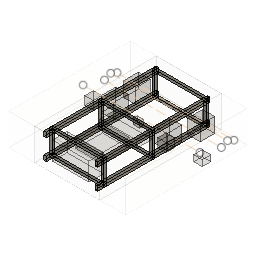
GP_TARS_V2_1000_CONCEPT_V0 (Autodesk Fusion 360 design; units mm, degrees)
part number: 2026-08-09-22-24-51-238
part number: 2026-08-09-22-24-51-360
part number: 2026-08-09-22-24-51-366
part number: 2026-08-09-22-24-51-368
part number: 2026-08-09-22-24-51-370
part number: 2026-08-09-22-24-51-373
part number: 2026-08-09-22-24-51-375
part number: 2026-08-09-22-24-51-377
part number: 2026-08-09-22-24-51-379
part number: 2026-08-09-22-24-51-381
part number: 2026-08-09-22-24-51-383
part number: 2026-08-09-22-24-51-385
part number: 2026-08-09-22-24-51-387
part number: 2026-08-09-22-24-51-390
part number: 2026-08-09-22-24-51-392
part number: 2026-08-09-22-24-51-395
part number: 2026-08-09-22-24-51-398
part number: 2026-08-09-22-24-51-400
part number: 2026-08-09-22-24-51-403
part number: 2026-08-09-22-24-51-405
part number: 2026-08-09-22-24-51-407
part number: 2026-08-09-22-24-51-410
part number: 2026-08-09-22-24-51-412
part number: 2026-08-09-22-24-51-415
part number: 2026-08-09-22-24-51-417
part number: 2026-08-09-22-24-51-420
part number: 2026-08-09-22-24-51-423
part number: 2026-08-09-22-24-51-426
part number: 2026-08-09-22-24-51-429
part number: 2026-08-09-22-24-51-432
part number: 2026-08-09-22-24-51-435
part number: 2026-08-09-22-24-51-438
part number: 2026-08-09-22-24-51-441
part number: 2026-08-09-22-24-51-444
part number: 2026-08-09-22-24-51-448
part number: 2026-08-09-22-24-51-451
part number: 2026-08-09-22-24-51-454
part number: 2026-08-09-22-24-51-459
part number: 2026-08-09-22-24-51-463
part number: 2026-08-09-22-24-51-467
part number: 2026-08-09-22-24-51-471
part number: 2026-08-09-22-24-51-475
part number: 2026-08-09-22-24-51-479
part number: 2026-08-09-22-24-51-483
part number: 2026-08-09-22-24-51-487
part number: 2026-08-09-22-24-51-492
part number: 2026-08-09-22-24-51-496
part number: 2026-08-09-22-24-51-501
part number: 2026-08-09-22-24-51-505
part number: 2026-08-09-22-24-51-510
part number: 2026-08-09-22-24-51-514
part number: 2026-08-09-22-24-51-519
part number: 2026-08-09-22-24-51-524
part number: 2026-08-09-22-24-51-612
part number: 2026-08-09-22-24-51-658
part number: 2026-08-09-22-24-51-683
part number: 2026-08-09-22-24-51-707
part number: 2026-08-09-22-24-51-732
part number: 2026-08-09-22-24-51-761
part number: 2026-08-09-22-24-51-801
part number: 2026-08-09-22-24-51-843
part number: 2026-08-09-22-24-51-883
part number: 2026-08-09-22-24-51-924
part number: 2026-08-09-22-24-51-965
part number: 2026-08-09-22-24-52-009
part number: 2026-08-09-22-24-52-056
part number: 2026-08-09-22-24-52-102
part number: 2026-08-09-22-24-52-148
part number: 2026-08-09-22-24-52-195
part number: 2026-08-09-22-24-52-243
part number: 2026-08-09-22-24-52-292
part number: 2026-08-09-22-24-52-342
part number: 2026-08-09-22-24-52-394
part number: 2026-08-09-22-24-52-450
part number: 2026-08-09-22-24-52-513
part number: 2026-08-09-22-24-52-576
part number: 2026-08-09-22-24-52-637
part number: 2026-08-09-22-24-52-701
part number: 2026-08-09-22-24-52-761
part number: 2026-08-09-22-24-52-825
part number: 2026-08-09-22-24-52-889
part number: 2026-08-09-22-24-52-958
part number: 2026-08-09-22-24-53-024
part number: 2026-08-09-22-24-53-092
part number: 2026-08-09-22-24-53-162
Autodesk Fusion 360 part; units mm, degrees
sketch "EXTERNAL_REFERENCE_ENVELOPE_PROFILE" plane through (0, 0, 0) normal (0, 0, 1) x (1, 0, 0) in component "EXTERNAL_REFERENCE_ENVELOPE"
  line L0 (-479.3589, 0) -> (479.3589, 0)
  line L1 (479.3589, 0) -> (479.3589, 1000)
  line L2 (479.3589, 1000) -> (-479.3589, 1000)
  line L3 (-479.3589, 1000) -> (-479.3589, 0)
extrude "Extrude1" add sketch "EXTERNAL_REFERENCE_ENVELOPE_PROFILE" along normal blind 259.8674 makes body 1 in component "EXTERNAL_REFERENCE_ENVELOPE"
move_body "Move1" bodies 1 to x (1, 0, 0) y (0, 1, 0) z (0, 0, 1) at (0, 0, -129.9337) in component "EXTERNAL_REFERENCE_ENVELOPE"
sketch "CENTRAL_CHASSIS_REFERENCE_PROFILE" plane through (0, 0, 0) normal (0, 0, 1) x (1, 0, 0) in component "CENTRAL_CHASSIS_REFERENCE"
  line L0 (-266.0414, 0) -> (266.0414, 0)
  line L1 (266.0414, 0) -> (266.0414, 998.6144)
  line L2 (266.0414, 998.6144) -> (-266.0414, 998.6144)
  line L3 (-266.0414, 998.6144) -> (-266.0414, 0)
extrude "Extrude1'" add sketch "CENTRAL_CHASSIS_REFERENCE_PROFILE" along normal blind 259.8674 separate body makes body 2 in component "CENTRAL_CHASSIS_REFERENCE"
move_body "Move1'" bodies 2 to x (1, 0, 0) y (0, 1, 0) z (0, 0, 1) at (0, 0, -129.9337) in component "CENTRAL_CHASSIS_REFERENCE"
ref_plane "WorkPlane1" through (0, 0, 0) normal (1, 0, 0) x (0, 1, 0) in component "DATUMS"
ref_plane "WorkPlane2" through (0, 0, 0) normal (0, 1, 0) x (0, 0, 1) in component "DATUMS"
ref_plane "WorkPlane3" through (0, 0, 0) normal (0, 0, 1) x (1, 0, 0) in component "DATUMS"
ref_plane "WorkPlane1" through (0, 0, -19.948) normal (0, 0, 1) x (1, 0, 0) in component "JOINT_UPPER_MAIN_REF"
sketch "JOINT_UPPER_MAIN_REF_AXIS_X" plane through (0, 0, -19.948) normal (0, 0, 1) x (1, 0, 0) in component "JOINT_UPPER_MAIN_REF"
  line L0 (-479.3589, 837.977) -> (479.3589, 837.977) construction
ref_plane "WorkPlane1" through (0, 0, -41.913) normal (0, 0, 1) x (1, 0, 0) in component "JOINT_UPPER_SECONDARY_REF"
sketch "JOINT_UPPER_SECONDARY_REF_AXIS_X" plane through (0, 0, -41.913) normal (0, 0, 1) x (1, 0, 0) in component "JOINT_UPPER_SECONDARY_REF"
  line L0 (-479.3589, 889.895) -> (479.3589, 889.895) construction
ref_plane "WorkPlane1" through (0, 0, -41.913) normal (0, 0, 1) x (1, 0, 0) in component "JOINT_LOWER_SECONDARY_REF"
sketch "JOINT_LOWER_SECONDARY_REF_AXIS_X" plane through (0, 0, -41.913) normal (0, 0, 1) x (1, 0, 0) in component "JOINT_LOWER_SECONDARY_REF"
  line L0 (-479.3589, 786.06) -> (479.3589, 786.06) construction
ref_plane "WorkPlane1" through (0, 0, 10.004) normal (0, 0, 1) x (1, 0, 0) in component "JOINT_LOWER_MAIN_REF"
sketch "JOINT_LOWER_MAIN_REF_AXIS_X" plane through (0, 0, 10.004) normal (0, 0, 1) x (1, 0, 0) in component "JOINT_LOWER_MAIN_REF"
  line L0 (-479.3589, 610.838) -> (479.3589, 610.838) construction
sketch "FRAME_VERTICAL_0_0_PROFILE" plane through (0, 0, 0) normal (0, 0, 1) x (1, 0, 0) in component "FRAME_VERTICAL_0_0"
  line L0 (-220, 30) -> (-200, 30)
  line L1 (-200, 30) -> (-200, 950)
  line L2 (-200, 950) -> (-220, 950)
  line L3 (-220, 950) -> (-220, 30)
extrude "Extrude1''" add sketch "FRAME_VERTICAL_0_0_PROFILE" along normal blind 40 separate body makes body 3 in component "FRAME_VERTICAL_0_0"
move_body "Move1''" bodies 3 to x (1, 0, 0) y (0, 1, 0) z (0, 0, 1) at (0, 0, -105) in component "FRAME_VERTICAL_0_0"
sketch "FRAME_VERTICAL_0_1_PROFILE" plane through (0, 0, 0) normal (0, 0, 1) x (1, 0, 0) in component "FRAME_VERTICAL_0_1"
  line L0 (-220, 30) -> (-200, 30)
  line L1 (-200, 30) -> (-200, 950)
  line L2 (-200, 950) -> (-220, 950)
  line L3 (-220, 950) -> (-220, 30)
extrude "Extrude1'''" add sketch "FRAME_VERTICAL_0_1_PROFILE" along normal blind 40 separate body makes body 4 in component "FRAME_VERTICAL_0_1"
move_body "Move1'''" bodies 4 to x (1, 0, 0) y (0, 1, 0) z (0, 0, 1) at (0, 0, 65) in component "FRAME_VERTICAL_0_1"
sketch "FRAME_VERTICAL_1_0_PROFILE" plane through (0, 0, 0) normal (0, 0, 1) x (1, 0, 0) in component "FRAME_VERTICAL_1_0"
  line L0 (200, 30) -> (220, 30)
  line L1 (220, 30) -> (220, 950)
  line L2 (220, 950) -> (200, 950)
  line L3 (200, 950) -> (200, 30)
extrude "Extrude1''''" add sketch "FRAME_VERTICAL_1_0_PROFILE" along normal blind 40 separate body makes body 5 in component "FRAME_VERTICAL_1_0"
move_body "Move1''''" bodies 5 to x (1, 0, 0) y (0, 1, 0) z (0, 0, 1) at (0, 0, -105) in component "FRAME_VERTICAL_1_0"
sketch "FRAME_VERTICAL_1_1_PROFILE" plane through (0, 0, 0) normal (0, 0, 1) x (1, 0, 0) in component "FRAME_VERTICAL_1_1"
  line L0 (200, 30) -> (220, 30)
  line L1 (220, 30) -> (220, 950)
  line L2 (220, 950) -> (200, 950)
  line L3 (200, 950) -> (200, 30)
extrude "Extrude1'''''" add sketch "FRAME_VERTICAL_1_1_PROFILE" along normal blind 40 separate body makes body 6 in component "FRAME_VERTICAL_1_1"
move_body "Move1'''''" bodies 6 to x (1, 0, 0) y (0, 1, 0) z (0, 0, 1) at (0, 0, 65) in component "FRAME_VERTICAL_1_1"
sketch "FRAME_CROSS_LOW_FRONT_PROFILE" plane through (0, 0, 0) normal (0, 0, 1) x (1, 0, 0) in component "FRAME_CROSS_LOW_FRONT"
  line L0 (-220, 80) -> (220, 80)
  line L1 (220, 80) -> (220, 100)
  line L2 (220, 100) -> (-220, 100)
  line L3 (-220, 100) -> (-220, 80)
extrude "Extrude1''''''" add sketch "FRAME_CROSS_LOW_FRONT_PROFILE" along normal blind 20 separate body makes body 7 in component "FRAME_CROSS_LOW_FRONT"
move_body "Move1''''''" bodies 7 to x (1, 0, 0) y (0, 1, 0) z (0, 0, 1) at (0, 0, -105) in component "FRAME_CROSS_LOW_FRONT"
sketch "FRAME_CROSS_LOW_REAR_PROFILE" plane through (0, 0, 0) normal (0, 0, 1) x (1, 0, 0) in component "FRAME_CROSS_LOW_REAR"
  line L0 (-220, 80) -> (220, 80)
  line L1 (220, 80) -> (220, 100)
  line L2 (220, 100) -> (-220, 100)
  line L3 (-220, 100) -> (-220, 80)
extrude "Extrude1'''''''" add sketch "FRAME_CROSS_LOW_REAR_PROFILE" along normal blind 20 separate body makes body 8 in component "FRAME_CROSS_LOW_REAR"
move_body "Move1'''''''" bodies 8 to x (1, 0, 0) y (0, 1, 0) z (0, 0, 1) at (0, 0, 85) in component "FRAME_CROSS_LOW_REAR"
sketch "FRAME_DEPTH_LOW_LEFT_PROFILE" plane through (0, 0, 0) normal (0, 0, 1) x (1, 0, 0) in component "FRAME_DEPTH_LOW_LEFT"
  line L0 (-220, 80) -> (-200, 80)
  line L1 (-200, 80) -> (-200, 100)
  line L2 (-200, 100) -> (-220, 100)
  line L3 (-220, 100) -> (-220, 80)
extrude "Extrude1''''''''" add sketch "FRAME_DEPTH_LOW_LEFT_PROFILE" along normal blind 170 separate body makes body 9 in component "FRAME_DEPTH_LOW_LEFT"
move_body "Move1''''''''" bodies 9 to x (1, 0, 0) y (0, 1, 0) z (0, 0, 1) at (0, 0, -85) in component "FRAME_DEPTH_LOW_LEFT"
sketch "FRAME_DEPTH_LOW_RIGHT_PROFILE" plane through (0, 0, 0) normal (0, 0, 1) x (1, 0, 0) in component "FRAME_DEPTH_LOW_RIGHT"
  line L0 (200, 80) -> (220, 80)
  line L1 (220, 80) -> (220, 100)
  line L2 (220, 100) -> (200, 100)
  line L3 (200, 100) -> (200, 80)
extrude "Extrude1'''''''''" add sketch "FRAME_DEPTH_LOW_RIGHT_PROFILE" along normal blind 170 separate body makes body 10 in component "FRAME_DEPTH_LOW_RIGHT"
move_body "Move1'''''''''" bodies 10 to x (1, 0, 0) y (0, 1, 0) z (0, 0, 1) at (0, 0, -85) in component "FRAME_DEPTH_LOW_RIGHT"
sketch "FRAME_CROSS_MID_FRONT_PROFILE" plane through (0, 0, 0) normal (0, 0, 1) x (1, 0, 0) in component "FRAME_CROSS_MID_FRONT"
  line L0 (-220, 480) -> (220, 480)
  line L1 (220, 480) -> (220, 500)
  line L2 (220, 500) -> (-220, 500)
  line L3 (-220, 500) -> (-220, 480)
extrude "Extrude1''''''''''" add sketch "FRAME_CROSS_MID_FRONT_PROFILE" along normal blind 20 separate body makes body 11 in component "FRAME_CROSS_MID_FRONT"
move_body "Move1''''''''''" bodies 11 to x (1, 0, 0) y (0, 1, 0) z (0, 0, 1) at (0, 0, -105) in component "FRAME_CROSS_MID_FRONT"
sketch "FRAME_CROSS_MID_REAR_PROFILE" plane through (0, 0, 0) normal (0, 0, 1) x (1, 0, 0) in component "FRAME_CROSS_MID_REAR"
  line L0 (-220, 480) -> (220, 480)
  line L1 (220, 480) -> (220, 500)
  line L2 (220, 500) -> (-220, 500)
  line L3 (-220, 500) -> (-220, 480)
extrude "Extrude1'''''''''''" add sketch "FRAME_CROSS_MID_REAR_PROFILE" along normal blind 20 separate body makes body 12 in component "FRAME_CROSS_MID_REAR"
move_body "Move1'''''''''''" bodies 12 to x (1, 0, 0) y (0, 1, 0) z (0, 0, 1) at (0, 0, 85) in component "FRAME_CROSS_MID_REAR"
sketch "FRAME_DEPTH_MID_LEFT_PROFILE" plane through (0, 0, 0) normal (0, 0, 1) x (1, 0, 0) in component "FRAME_DEPTH_MID_LEFT"
  line L0 (-220, 480) -> (-200, 480)
  line L1 (-200, 480) -> (-200, 500)
  line L2 (-200, 500) -> (-220, 500)
  line L3 (-220, 500) -> (-220, 480)
extrude "Extrude1''''''''''''" add sketch "FRAME_DEPTH_MID_LEFT_PROFILE" along normal blind 170 separate body makes body 13 in component "FRAME_DEPTH_MID_LEFT"
move_body "Move1''''''''''''" bodies 13 to x (1, 0, 0) y (0, 1, 0) z (0, 0, 1) at (0, 0, -85) in component "FRAME_DEPTH_MID_LEFT"
sketch "FRAME_DEPTH_MID_RIGHT_PROFILE" plane through (0, 0, 0) normal (0, 0, 1) x (1, 0, 0) in component "FRAME_DEPTH_MID_RIGHT"
  line L0 (200, 480) -> (220, 480)
  line L1 (220, 480) -> (220, 500)
  line L2 (220, 500) -> (200, 500)
  line L3 (200, 500) -> (200, 480)
extrude "Extrude1'''''''''''''" add sketch "FRAME_DEPTH_MID_RIGHT_PROFILE" along normal blind 170 separate body makes body 14 in component "FRAME_DEPTH_MID_RIGHT"
move_body "Move1'''''''''''''" bodies 14 to x (1, 0, 0) y (0, 1, 0) z (0, 0, 1) at (0, 0, -85) in component "FRAME_DEPTH_MID_RIGHT"
sketch "FRAME_CROSS_HIGH_FRONT_PROFILE" plane through (0, 0, 0) normal (0, 0, 1) x (1, 0, 0) in component "FRAME_CROSS_HIGH_FRONT"
  line L0 (-220, 920) -> (220, 920)
  line L1 (220, 920) -> (220, 940)
  line L2 (220, 940) -> (-220, 940)
  line L3 (-220, 940) -> (-220, 920)
extrude "Extrude1''''''''''''''" add sketch "FRAME_CROSS_HIGH_FRONT_PROFILE" along normal blind 20 separate body makes body 15 in component "FRAME_CROSS_HIGH_FRONT"
move_body "Move1''''''''''''''" bodies 15 to x (1, 0, 0) y (0, 1, 0) z (0, 0, 1) at (0, 0, -105) in component "FRAME_CROSS_HIGH_FRONT"
sketch "FRAME_CROSS_HIGH_REAR_PROFILE" plane through (0, 0, 0) normal (0, 0, 1) x (1, 0, 0) in component "FRAME_CROSS_HIGH_REAR"
  line L0 (-220, 920) -> (220, 920)
  line L1 (220, 920) -> (220, 940)
  line L2 (220, 940) -> (-220, 940)
  line L3 (-220, 940) -> (-220, 920)
extrude "Extrude1'''''''''''''''" add sketch "FRAME_CROSS_HIGH_REAR_PROFILE" along normal blind 20 separate body makes body 16 in component "FRAME_CROSS_HIGH_REAR"
move_body "Move1'''''''''''''''" bodies 16 to x (1, 0, 0) y (0, 1, 0) z (0, 0, 1) at (0, 0, 85) in component "FRAME_CROSS_HIGH_REAR"
sketch "FRAME_DEPTH_HIGH_LEFT_PROFILE" plane through (0, 0, 0) normal (0, 0, 1) x (1, 0, 0) in component "FRAME_DEPTH_HIGH_LEFT"
  line L0 (-220, 920) -> (-200, 920)
  line L1 (-200, 920) -> (-200, 940)
  line L2 (-200, 940) -> (-220, 940)
  line L3 (-220, 940) -> (-220, 920)
extrude "Extrude1''''''''''''''''" add sketch "FRAME_DEPTH_HIGH_LEFT_PROFILE" along normal blind 170 separate body makes body 17 in component "FRAME_DEPTH_HIGH_LEFT"
move_body "Move1''''''''''''''''" bodies 17 to x (1, 0, 0) y (0, 1, 0) z (0, 0, 1) at (0, 0, -85) in component "FRAME_DEPTH_HIGH_LEFT"
sketch "FRAME_DEPTH_HIGH_RIGHT_PROFILE" plane through (0, 0, 0) normal (0, 0, 1) x (1, 0, 0) in component "FRAME_DEPTH_HIGH_RIGHT"
  line L0 (200, 920) -> (220, 920)
  line L1 (220, 920) -> (220, 940)
  line L2 (220, 940) -> (200, 940)
  line L3 (200, 940) -> (200, 920)
extrude "Extrude1'''''''''''''''''" add sketch "FRAME_DEPTH_HIGH_RIGHT_PROFILE" along normal blind 170 separate body makes body 18 in component "FRAME_DEPTH_HIGH_RIGHT"
move_body "Move1'''''''''''''''''" bodies 18 to x (1, 0, 0) y (0, 1, 0) z (0, 0, 1) at (0, 0, -85) in component "FRAME_DEPTH_HIGH_RIGHT"
sketch "BATTERY_KEEP_OUT_PROFILE" plane through (0, 0, 0) normal (0, 0, 1) x (1, 0, 0) in component "BATTERY_KEEP_OUT"
  line L0 (-150, 30) -> (150, 30)
  line L1 (150, 30) -> (150, 150)
  line L2 (150, 150) -> (-150, 150)
  line L3 (-150, 150) -> (-150, 30)
extrude "Extrude1''''''''''''''''''" add sketch "BATTERY_KEEP_OUT_PROFILE" along normal blind 150 separate body makes body 19 in component "BATTERY_KEEP_OUT"
move_body "Move1''''''''''''''''''" bodies 19 to x (1, 0, 0) y (0, 1, 0) z (0, 0, 1) at (0, 0, -75) in component "BATTERY_KEEP_OUT"
sketch "MINI_PC_KEEP_OUT_PROFILE" plane through (0, 0, 0) normal (0, 0, 1) x (1, 0, 0) in component "MINI_PC_KEEP_OUT"
  line L0 (-110, 180) -> (110, 180)
  line L1 (110, 180) -> (110, 400)
  line L2 (110, 400) -> (-110, 400)
  line L3 (-110, 400) -> (-110, 180)
extrude "Extrude1'''''''''''''''''''" add sketch "MINI_PC_KEEP_OUT_PROFILE" along normal blind 80 separate body makes body 20 in component "MINI_PC_KEEP_OUT"
move_body "Move1'''''''''''''''''''" bodies 20 to x (1, 0, 0) y (0, 1, 0) z (0, 0, 1) at (0, 0, -40) in component "MINI_PC_KEEP_OUT"
sketch "GPU_KEEP_OUT_PROFILE" plane through (0, 0, 0) normal (0, 0, 1) x (1, 0, 0) in component "GPU_KEEP_OUT"
  line L0 (-150, 420) -> (150, 420)
  line L1 (150, 420) -> (150, 550)
  line L2 (150, 550) -> (-150, 550)
  line L3 (-150, 550) -> (-150, 420)
extrude "Extrude1''''''''''''''''''''" add sketch "GPU_KEEP_OUT_PROFILE" along normal blind 60 separate body makes body 21 in component "GPU_KEEP_OUT"
move_body "Move1''''''''''''''''''''" bodies 21 to x (1, 0, 0) y (0, 1, 0) z (0, 0, 1) at (0, 0, -30) in component "GPU_KEEP_OUT"
sketch "ACTUATOR_MAIN_UPPER_PORT_KEEP_OUT_PROFILE" plane through (0, 0, 0) normal (0, 0, 1) x (1, 0, 0) in component "ACTUATOR_MAIN_UPPER_PORT_KEEP_OUT"
  line L0 (214.041, 777.973) -> (314.041, 777.973)
  line L1 (314.041, 777.973) -> (314.041, 897.973)
  line L2 (314.041, 897.973) -> (214.041, 897.973)
  line L3 (214.041, 897.973) -> (214.041, 777.973)
extrude "Extrude1'''''''''''''''''''''" add sketch "ACTUATOR_MAIN_UPPER_PORT_KEEP_OUT_PROFILE" along normal blind 120 separate body makes body 22 in component "ACTUATOR_MAIN_UPPER_PORT_KEEP_OUT"
move_body "Move1'''''''''''''''''''''" bodies 22 to x (1, 0, 0) y (0, 1, 0) z (0, 0, 1) at (0, 0, -79.977) in component "ACTUATOR_MAIN_UPPER_PORT_KEEP_OUT"
sketch "ACTUATOR_MAIN_UPPER_STARBOARD_KEEP_OUT_PROFILE" plane through (0, 0, 0) normal (0, 0, 1) x (1, 0, 0) in component "ACTUATOR_MAIN_UPPER_STARBOARD_KEEP_OUT"
  line L0 (-314.041, 777.973) -> (-214.041, 777.973)
  line L1 (-214.041, 777.973) -> (-214.041, 897.973)
  line L2 (-214.041, 897.973) -> (-314.041, 897.973)
  line L3 (-314.041, 897.973) -> (-314.041, 777.973)
extrude "Extrude1''''''''''''''''''''''" add sketch "ACTUATOR_MAIN_UPPER_STARBOARD_KEEP_OUT_PROFILE" along normal blind 120 separate body makes body 23 in component "ACTUATOR_MAIN_UPPER_STARBOARD_KEEP_OUT"
move_body "Move1''''''''''''''''''''''" bodies 23 to x (1, 0, 0) y (0, 1, 0) z (0, 0, 1) at (0, 0, -79.977) in component "ACTUATOR_MAIN_UPPER_STARBOARD_KEEP_OUT"
sketch "ACTUATOR_MAIN_LOWER_PORT_KEEP_OUT_PROFILE" plane through (0, 0, 0) normal (0, 0, 1) x (1, 0, 0) in component "ACTUATOR_MAIN_LOWER_PORT_KEEP_OUT"
  line L0 (170, 550.838) -> (270, 550.838)
  line L1 (270, 550.838) -> (270, 670.838)
  line L2 (270, 670.838) -> (170, 670.838)
  line L3 (170, 670.838) -> (170, 550.838)
extrude "Extrude1'''''''''''''''''''''''" add sketch "ACTUATOR_MAIN_LOWER_PORT_KEEP_OUT_PROFILE" along normal blind 120 separate body makes body 24 in component "ACTUATOR_MAIN_LOWER_PORT_KEEP_OUT"
move_body "Move1'''''''''''''''''''''''" bodies 24 to x (1, 0, 0) y (0, 1, 0) z (0, 0, 1) at (0, 0, -49.996) in component "ACTUATOR_MAIN_LOWER_PORT_KEEP_OUT"
sketch "ACTUATOR_MAIN_LOWER_STARBOARD_KEEP_OUT_PROFILE" plane through (0, 0, 0) normal (0, 0, 1) x (1, 0, 0) in component "ACTUATOR_MAIN_LOWER_STARBOARD_KEEP_OUT"
  line L0 (-270, 550.838) -> (-170, 550.838)
  line L1 (-170, 550.838) -> (-170, 670.838)
  line L2 (-170, 670.838) -> (-270, 670.838)
  line L3 (-270, 670.838) -> (-270, 550.838)
extrude "Extrude1''''''''''''''''''''''''" add sketch "ACTUATOR_MAIN_LOWER_STARBOARD_KEEP_OUT_PROFILE" along normal blind 120 separate body makes body 25 in component "ACTUATOR_MAIN_LOWER_STARBOARD_KEEP_OUT"
move_body "Move1''''''''''''''''''''''''" bodies 25 to x (1, 0, 0) y (0, 1, 0) z (0, 0, 1) at (0, 0, -49.996) in component "ACTUATOR_MAIN_LOWER_STARBOARD_KEEP_OUT"
sketch "ACTUATOR_SECONDARY_PORT_KEEP_OUT_PROFILE" plane through (0, 0, 0) normal (0, 0, 1) x (1, 0, 0) in component "ACTUATOR_SECONDARY_PORT_KEEP_OUT"
  line L0 (264.185, 479.664) -> (334.185, 479.664)
  line L1 (334.185, 479.664) -> (334.185, 549.664)
  line L2 (334.185, 549.664) -> (264.185, 549.664)
  line L3 (264.185, 549.664) -> (264.185, 479.664)
extrude "Extrude1'''''''''''''''''''''''''" add sketch "ACTUATOR_SECONDARY_PORT_KEEP_OUT_PROFILE" along normal blind 70 separate body makes body 26 in component "ACTUATOR_SECONDARY_PORT_KEEP_OUT"
move_body "Move1'''''''''''''''''''''''''" bodies 26 to x (1, 0, 0) y (0, 1, 0) z (0, 0, 1) at (0, 0, 2.955) in component "ACTUATOR_SECONDARY_PORT_KEEP_OUT"
sketch "ACTUATOR_SECONDARY_STARBOARD_KEEP_OUT_PROFILE" plane through (0, 0, 0) normal (0, 0, 1) x (1, 0, 0) in component "ACTUATOR_SECONDARY_STARBOARD_KEEP_OUT"
  line L0 (-334.185, 479.664) -> (-264.185, 479.664)
  line L1 (-264.185, 479.664) -> (-264.185, 549.664)
  line L2 (-264.185, 549.664) -> (-334.185, 549.664)
  line L3 (-334.185, 549.664) -> (-334.185, 479.664)
extrude "Extrude1''''''''''''''''''''''''''" add sketch "ACTUATOR_SECONDARY_STARBOARD_KEEP_OUT_PROFILE" along normal blind 70 separate body makes body 27 in component "ACTUATOR_SECONDARY_STARBOARD_KEEP_OUT"
move_body "Move1''''''''''''''''''''''''''" bodies 27 to x (1, 0, 0) y (0, 1, 0) z (0, 0, 1) at (0, 0, 2.955) in component "ACTUATOR_SECONDARY_STARBOARD_KEEP_OUT"
sketch "E_STOP_KEEP_OUT_PROFILE" plane through (0, 0, 0) normal (0, 0, 1) x (1, 0, 0) in component "E_STOP_KEEP_OUT"
  line L0 (389.3589, 650) -> (459.3589, 650)
  line L1 (459.3589, 650) -> (459.3589, 720)
  line L2 (459.3589, 720) -> (389.3589, 720)
  line L3 (389.3589, 720) -> (389.3589, 650)
extrude "Extrude1'''''''''''''''''''''''''''" add sketch "E_STOP_KEEP_OUT_PROFILE" along normal blind 50 separate body makes body 28 in component "E_STOP_KEEP_OUT"
move_body "Move1'''''''''''''''''''''''''''" bodies 28 to x (1, 0, 0) y (0, 1, 0) z (0, 0, 1) at (0, 0, -119.9337) in component "E_STOP_KEEP_OUT"
sketch "IMU_KEEP_OUT_PROFILE" plane through (0, 0, 0) normal (0, 0, 1) x (1, 0, 0) in component "IMU_KEEP_OUT"
  line L0 (-25, 570) -> (25, 570)
  line L1 (25, 570) -> (25, 600)
  line L2 (25, 600) -> (-25, 600)
  line L3 (-25, 600) -> (-25, 570)
extrude "Extrude1''''''''''''''''''''''''''''" add sketch "IMU_KEEP_OUT_PROFILE" along normal blind 50 separate body makes body 29 in component "IMU_KEEP_OUT"
move_body "Move1''''''''''''''''''''''''''''" bodies 29 to x (1, 0, 0) y (0, 1, 0) z (0, 0, 1) at (0, 0, -25) in component "IMU_KEEP_OUT"
component "00_MASTER_REFERENCE" placed x (1, 0, 0) y (0, 1, 0) z (0, 0, 1) at (0, 0, 0)
component "01_FRAME" placed x (1, 0, 0) y (0, 1, 0) z (0, 0, 1) at (0, 0, 0)
component "02_JOINTS" placed x (1, 0, 0) y (0, 1, 0) z (0, 0, 1) at (0, 0, 0)
component "03_ACTUATORS" placed x (1, 0, 0) y (0, 1, 0) z (0, 0, 1) at (0, 0, 0)
component "04_BEARINGS_SHAFTS" placed x (1, 0, 0) y (0, 1, 0) z (0, 0, 1) at (0, 0, 0)
component "05_BATTERY" placed x (1, 0, 0) y (0, 1, 0) z (0, 0, 1) at (0, 0, 0)
component "06_COMPUTE" placed x (1, 0, 0) y (0, 1, 0) z (0, 0, 1) at (0, 0, 0)
component "07_GPU" placed x (1, 0, 0) y (0, 1, 0) z (0, 0, 1) at (0, 0, 0)
component "08_ELECTRONICS" placed x (1, 0, 0) y (0, 1, 0) z (0, 0, 1) at (0, 0, 0)
component "09_COOLING" placed x (1, 0, 0) y (0, 1, 0) z (0, 0, 1) at (0, 0, 0)
component "10_SENSORS" placed x (1, 0, 0) y (0, 1, 0) z (0, 0, 1) at (0, 0, 0)
component "11_BODY_PANELS" placed x (1, 0, 0) y (0, 1, 0) z (0, 0, 1) at (0, 0, 0)
component "12_FASTENERS" placed x (1, 0, 0) y (0, 1, 0) z (0, 0, 1) at (0, 0, 0)
component "13_WIRING" placed x (1, 0, 0) y (0, 1, 0) z (0, 0, 1) at (0, 0, 0)
component "Original_1000mm_Scaled_Geometry" placed x (1, 0, 0) y (0, 1, 0) z (0, 0, 1) at (0, 0, 0) in component "00_MASTER_REFERENCE"
component "DATUMS" placed x (1, 0, 0) y (0, 1, 0) z (0, 0, 1) at (0, 0, 0) in component "00_MASTER_REFERENCE"
component "Central_Spine" placed x (1, 0, 0) y (0, 1, 0) z (0, 0, 1) at (0, 0, 0) in component "01_FRAME"
component "Left_Frame" placed x (1, 0, 0) y (0, 1, 0) z (0, 0, 1) at (0, 0, 0) in component "01_FRAME"
component "Right_Frame" placed x (1, 0, 0) y (0, 1, 0) z (0, 0, 1) at (0, 0, 0) in component "01_FRAME"
component "Crossmembers" placed x (1, 0, 0) y (0, 1, 0) z (0, 0, 1) at (0, 0, 0) in component "01_FRAME"
component "FRAME_VERTICAL_0_0" placed x (1, 0, 0) y (0, 1, 0) z (0, 0, 1) at (0, 0, 0) in component "01_FRAME"
component "FRAME_VERTICAL_0_1" placed x (1, 0, 0) y (0, 1, 0) z (0, 0, 1) at (0, 0, 0) in component "01_FRAME"
component "FRAME_VERTICAL_1_0" placed x (1, 0, 0) y (0, 1, 0) z (0, 0, 1) at (0, 0, 0) in component "01_FRAME"
component "FRAME_VERTICAL_1_1" placed x (1, 0, 0) y (0, 1, 0) z (0, 0, 1) at (0, 0, 0) in component "01_FRAME"
component "FRAME_CROSS_LOW_FRONT" placed x (1, 0, 0) y (0, 1, 0) z (0, 0, 1) at (0, 0, 0) in component "01_FRAME"
component "FRAME_CROSS_LOW_REAR" placed x (1, 0, 0) y (0, 1, 0) z (0, 0, 1) at (0, 0, 0) in component "01_FRAME"
component "FRAME_DEPTH_LOW_LEFT" placed x (1, 0, 0) y (0, 1, 0) z (0, 0, 1) at (0, 0, 0) in component "01_FRAME"
component "FRAME_DEPTH_LOW_RIGHT" placed x (1, 0, 0) y (0, 1, 0) z (0, 0, 1) at (0, 0, 0) in component "01_FRAME"
component "FRAME_CROSS_MID_FRONT" placed x (1, 0, 0) y (0, 1, 0) z (0, 0, 1) at (0, 0, 0) in component "01_FRAME"
component "FRAME_CROSS_MID_REAR" placed x (1, 0, 0) y (0, 1, 0) z (0, 0, 1) at (0, 0, 0) in component "01_FRAME"
component "FRAME_DEPTH_MID_LEFT" placed x (1, 0, 0) y (0, 1, 0) z (0, 0, 1) at (0, 0, 0) in component "01_FRAME"
component "FRAME_DEPTH_MID_RIGHT" placed x (1, 0, 0) y (0, 1, 0) z (0, 0, 1) at (0, 0, 0) in component "01_FRAME"
component "FRAME_CROSS_HIGH_FRONT" placed x (1, 0, 0) y (0, 1, 0) z (0, 0, 1) at (0, 0, 0) in component "01_FRAME"
component "FRAME_CROSS_HIGH_REAR" placed x (1, 0, 0) y (0, 1, 0) z (0, 0, 1) at (0, 0, 0) in component "01_FRAME"
component "FRAME_DEPTH_HIGH_LEFT" placed x (1, 0, 0) y (0, 1, 0) z (0, 0, 1) at (0, 0, 0) in component "01_FRAME"
component "FRAME_DEPTH_HIGH_RIGHT" placed x (1, 0, 0) y (0, 1, 0) z (0, 0, 1) at (0, 0, 0) in component "01_FRAME"
component "Upper_Pivot" placed x (1, 0, 0) y (0, 1, 0) z (0, 0, 1) at (0, 0, 0) in component "02_JOINTS"
component "Lower_Pivot" placed x (1, 0, 0) y (0, 1, 0) z (0, 0, 1) at (0, 0, 0) in component "02_JOINTS"
component "Left_Leg_Pivot" placed x (1, 0, 0) y (0, 1, 0) z (0, 0, 1) at (0, 0, 0) in component "02_JOINTS"
component "Right_Leg_Pivot" placed x (1, 0, 0) y (0, 1, 0) z (0, 0, 1) at (0, 0, 0) in component "02_JOINTS"
component "JOINT_UPPER_MAIN_REF" placed x (1, 0, 0) y (0, 1, 0) z (0, 0, 1) at (0, 0, 0) in component "02_JOINTS"
component "JOINT_UPPER_SECONDARY_REF" placed x (1, 0, 0) y (0, 1, 0) z (0, 0, 1) at (0, 0, 0) in component "02_JOINTS"
component "JOINT_LOWER_SECONDARY_REF" placed x (1, 0, 0) y (0, 1, 0) z (0, 0, 1) at (0, 0, 0) in component "02_JOINTS"
component "JOINT_LOWER_MAIN_REF" placed x (1, 0, 0) y (0, 1, 0) z (0, 0, 1) at (0, 0, 0) in component "02_JOINTS"
component "ACTUATOR_MAIN_PLACEHOLDERS" placed x (1, 0, 0) y (0, 1, 0) z (0, 0, 1) at (0, 0, 0) in component "03_ACTUATORS"
component "ACTUATOR_SECONDARY_PLACEHOLDERS" placed x (1, 0, 0) y (0, 1, 0) z (0, 0, 1) at (0, 0, 0) in component "03_ACTUATORS"
component "ACTUATOR_MAIN_UPPER_PORT_KEEP_OUT" placed x (1, 0, 0) y (0, 1, 0) z (0, 0, 1) at (0, 0, 0) in component "03_ACTUATORS"
component "ACTUATOR_MAIN_UPPER_STARBOARD_KEEP_OUT" placed x (1, 0, 0) y (0, 1, 0) z (0, 0, 1) at (0, 0, 0) in component "03_ACTUATORS"
component "ACTUATOR_MAIN_LOWER_PORT_KEEP_OUT" placed x (1, 0, 0) y (0, 1, 0) z (0, 0, 1) at (0, 0, 0) in component "03_ACTUATORS"
component "ACTUATOR_MAIN_LOWER_STARBOARD_KEEP_OUT" placed x (1, 0, 0) y (0, 1, 0) z (0, 0, 1) at (0, 0, 0) in component "03_ACTUATORS"
component "ACTUATOR_SECONDARY_PORT_KEEP_OUT" placed x (1, 0, 0) y (0, 1, 0) z (0, 0, 1) at (0, 0, 0) in component "03_ACTUATORS"
component "ACTUATOR_SECONDARY_STARBOARD_KEEP_OUT" placed x (1, 0, 0) y (0, 1, 0) z (0, 0, 1) at (0, 0, 0) in component "03_ACTUATORS"
component "MAIN_SHAFTS" placed x (1, 0, 0) y (0, 1, 0) z (0, 0, 1) at (0, 0, 0) in component "04_BEARINGS_SHAFTS"
component "SECONDARY_SHAFTS" placed x (1, 0, 0) y (0, 1, 0) z (0, 0, 1) at (0, 0, 0) in component "04_BEARINGS_SHAFTS"
component "BATTERY_TRAY_PLACEHOLDER" placed x (1, 0, 0) y (0, 1, 0) z (0, 0, 1) at (0, 0, 0) in component "05_BATTERY"
component "BATTERY_KEEP_OUT" placed x (1, 0, 0) y (0, 1, 0) z (0, 0, 1) at (0, 0, 0) in component "05_BATTERY"
component "MINI_PC_TRAY_PLACEHOLDER" placed x (1, 0, 0) y (0, 1, 0) z (0, 0, 1) at (0, 0, 0) in component "06_COMPUTE"
component "MINI_PC_KEEP_OUT" placed x (1, 0, 0) y (0, 1, 0) z (0, 0, 1) at (0, 0, 0) in component "06_COMPUTE"
component "GPU_BRACKET_PLACEHOLDER" placed x (1, 0, 0) y (0, 1, 0) z (0, 0, 1) at (0, 0, 0) in component "07_GPU"
component "GPU_KEEP_OUT" placed x (1, 0, 0) y (0, 1, 0) z (0, 0, 1) at (0, 0, 0) in component "07_GPU"
component "MOTOR_CONTROLLER" placed x (1, 0, 0) y (0, 1, 0) z (0, 0, 1) at (0, 0, 0) in component "08_ELECTRONICS"
component "CAN_INTERFACE" placed x (1, 0, 0) y (0, 1, 0) z (0, 0, 1) at (0, 0, 0) in component "08_ELECTRONICS"
component "POWER_DISTRIBUTION" placed x (1, 0, 0) y (0, 1, 0) z (0, 0, 1) at (0, 0, 0) in component "08_ELECTRONICS"
component "SAFETY_CONTROLLER" placed x (1, 0, 0) y (0, 1, 0) z (0, 0, 1) at (0, 0, 0) in component "08_ELECTRONICS"
component "E_STOP_KEEP_OUT" placed x (1, 0, 0) y (0, 1, 0) z (0, 0, 1) at (0, 0, 0) in component "08_ELECTRONICS"
component "LOW_INTAKE" placed x (1, 0, 0) y (0, 1, 0) z (0, 0, 1) at (0, 0, 0) in component "09_COOLING"
component "GPU_AIR_PATH" placed x (1, 0, 0) y (0, 1, 0) z (0, 0, 1) at (0, 0, 0) in component "09_COOLING"
component "COMPUTE_AIR_PATH" placed x (1, 0, 0) y (0, 1, 0) z (0, 0, 1) at (0, 0, 0) in component "09_COOLING"
component "HIGH_EXHAUST" placed x (1, 0, 0) y (0, 1, 0) z (0, 0, 1) at (0, 0, 0) in component "09_COOLING"
component "IMU" placed x (1, 0, 0) y (0, 1, 0) z (0, 0, 1) at (0, 0, 0) in component "10_SENSORS"
component "RGB_CAMERA" placed x (1, 0, 0) y (0, 1, 0) z (0, 0, 1) at (0, 0, 0) in component "10_SENSORS"
component "DEPTH_CAMERA" placed x (1, 0, 0) y (0, 1, 0) z (0, 0, 1) at (0, 0, 0) in component "10_SENSORS"
component "MIC_ARRAY" placed x (1, 0, 0) y (0, 1, 0) z (0, 0, 1) at (0, 0, 0) in component "10_SENSORS"
component "GROUND_CONTACT" placed x (1, 0, 0) y (0, 1, 0) z (0, 0, 1) at (0, 0, 0) in component "10_SENSORS"
component "OPTIONAL_LIDAR" placed x (1, 0, 0) y (0, 1, 0) z (0, 0, 1) at (0, 0, 0) in component "10_SENSORS"
component "IMU_KEEP_OUT" placed x (1, 0, 0) y (0, 1, 0) z (0, 0, 1) at (0, 0, 0) in component "10_SENSORS"
component "COMPUTE_ACCESS" placed x (1, 0, 0) y (0, 1, 0) z (0, 0, 1) at (0, 0, 0) in component "11_BODY_PANELS"
component "GPU_ACCESS" placed x (1, 0, 0) y (0, 1, 0) z (0, 0, 1) at (0, 0, 0) in component "11_BODY_PANELS"
component "BATTERY_ACCESS" placed x (1, 0, 0) y (0, 1, 0) z (0, 0, 1) at (0, 0, 0) in component "11_BODY_PANELS"
component "MOTOR_CONTROLLER_ACCESS" placed x (1, 0, 0) y (0, 1, 0) z (0, 0, 1) at (0, 0, 0) in component "11_BODY_PANELS"
component "LEFT_ACTUATOR_ACCESS" placed x (1, 0, 0) y (0, 1, 0) z (0, 0, 1) at (0, 0, 0) in component "11_BODY_PANELS"
component "RIGHT_ACTUATOR_ACCESS" placed x (1, 0, 0) y (0, 1, 0) z (0, 0, 1) at (0, 0, 0) in component "11_BODY_PANELS"
component "EXTERNAL_REFERENCE_ENVELOPE" placed x (1, 0, 0) y (0, 1, 0) z (0, 0, 1) at (0, 0, 0) in component "Original_1000mm_Scaled_Geometry"
component "CENTRAL_CHASSIS_REFERENCE" placed x (1, 0, 0) y (0, 1, 0) z (0, 0, 1) at (0, 0, 0) in component "Original_1000mm_Scaled_Geometry"
equation "ROBOT_HEIGHT = 1000 mm" comment "Target standing height"
equation "SOURCE_HEIGHT = 250.3969610849432 mm" comment "Measured STEP height"
equation "REFERENCE_SCALE = ROBOT_HEIGHT / SOURCE_HEIGHT" comment "Reference only"
equation "ROBOT_WIDTH = 240.06 mm * REFERENCE_SCALE"
equation "ROBOT_DEPTH = 65.070011622468 mm * REFERENCE_SCALE"
equation "SHELL_WALL = 3 mm"
equation "FRAME_PROFILE_SMALL = 20 mm"
equation "FRAME_PROFILE_LARGE_X = 20 mm"
equation "FRAME_PROFILE_LARGE_Y = 40 mm"
equation "MAIN_SHAFT_DIAMETER = 20 mm"
equation "SECONDARY_SHAFT_DIAMETER = 12 mm"
equation "BATTERY_VOLTAGE = 24 V"
equation "GROUND_CLEARANCE = 20 mm"
equation "MINI_PC_X = 220 mm"
equation "MINI_PC_Y = 220 mm"
equation "MINI_PC_Z = 80 mm"
equation "GPU_LENGTH = 300 mm"
equation "GPU_HEIGHT = 130 mm"
equation "GPU_WIDTH = 60 mm"
equation "BATTERY_X = 300 mm"
equation "BATTERY_Y = 120 mm"
equation "BATTERY_Z = 150 mm"
equation "ACTUATOR_MAIN_D = 120 mm"
equation "ACTUATOR_MAIN_L = 100 mm"
equation "ACTUATOR_SECONDARY_D = 70 mm"
equation "ACTUATOR_SECONDARY_L = 70 mm"
named bodies: "EXTERNAL_REFERENCE_ENVELOPE", "CENTRAL_CHASSIS_REFERENCE", "FRAME_VERTICAL_0_0", "FRAME_VERTICAL_0_1", "FRAME_VERTICAL_1_0", "FRAME_VERTICAL_1_1", "FRAME_CROSS_LOW_FRONT", "FRAME_CROSS_LOW_REAR", "FRAME_DEPTH_LOW_LEFT", "FRAME_DEPTH_LOW_RIGHT", "FRAME_CROSS_MID_FRONT", "FRAME_CROSS_MID_REAR", "FRAME_DEPTH_MID_LEFT", "FRAME_DEPTH_MID_RIGHT", "FRAME_CROSS_HIGH_FRONT", "FRAME_CROSS_HIGH_REAR", "FRAME_DEPTH_HIGH_LEFT", "FRAME_DEPTH_HIGH_RIGHT", "BATTERY_KEEP_OUT", "MINI_PC_KEEP_OUT", "GPU_KEEP_OUT", "ACTUATOR_MAIN_UPPER_PORT_KEEP_OUT", "ACTUATOR_MAIN_UPPER_STARBOARD_KEEP_OUT", "ACTUATOR_MAIN_LOWER_PORT_KEEP_OUT", "ACTUATOR_MAIN_LOWER_STARBOARD_KEEP_OUT", "ACTUATOR_SECONDARY_PORT_KEEP_OUT", "ACTUATOR_SECONDARY_STARBOARD_KEEP_OUT", "E_STOP_KEEP_OUT", "IMU_KEEP_OUT"
